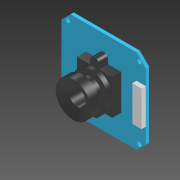
# Autodesk Inventor part: Arducam
Saved by Autodesk Inventor 2020 (Build 240168000, 168)
## iProperties
Created: 2020-11-17
Part Number: Arducam
Material: Generic
Document SubType Name: Modeling
Designer: valer
Density: 1 g/cm^3
Appearance: Default
Author: valer
Autodesk Inventor part; units mm, degrees
sketch "Base" plane through (0, 0, 0) normal (0, 0, 1) x (1, 0, 0)
  line L0 (-20.125, 20.125) -> (20.125, 20.125)
  line L1 (20.125, 20.125) -> (20.125, -20.125)
  line L2 (20.125, -20.125) -> (-20.125, -20.125)
  line L3 (-20.125, -20.125) -> (-20.125, 20.125)
  line L4 (-15.74, 20.125) -> (-20.125, 15.74)
  line L5 (15.74, 20.125) -> (20.125, 15.74)
  line L6 (-17.02, 17.02) -> (17.02, 17.02) construction
  line L7 (17.02, 17.02) -> (17.02, -17.02) construction
  line L8 (17.02, -17.02) -> (-17.02, -17.02) construction
  line L9 (-17.02, -17.02) -> (-17.02, 17.02) construction
  line L10 (-17.02, 17.02) -> (17.02, -17.02) construction
  line L11 (17.02, 17.02) -> (-17.02, -17.02) construction
  circle A0 centre (0, 0) radius 8.4
  circle A1 centre (17.02, 17.02) radius 1.05
  circle A2 centre (-17.02, 17.02) radius 1.05
  circle A3 centre (-17.02, -17.02) radius 1.05
  circle A4 centre (17.02, -17.02) radius 1.05
  line L12 (-20.125, -15.74) -> (-15.74, -20.125)
  line L13 (20.125, -15.74) -> (15.74, -20.125)
  point P0 (0, 0)
  point P1 (0, 0)
  dimension "d0" = 40.25
  dimension "d1" = 40.25
  dimension "d2" = 135
  dimension "d3" = 135
  dimension "d4" = 31.48
  dimension "d5" = 34.04
  dimension "d6" = 3.105
  dimension "d7" = 3.105
  dimension "d8" = 3.105
  dimension "d9" = 3.105
  dimension "d10" = 16.8
  dimension "d11" = 2.1
  dimension "d12" = 135
  dimension "d13" = 135
  dimension "d14" = 31.48
  dimension "d15" = 34.04
  dimension "d16" = 31.48
  constraints: 28 end point, 8 point on line, 5 centre point, 5 coincident, 5 perpendicular, 4 parallel, 3 equal radius, 2 horizontal, 2 midpoint
  measures "d0" distance of L0.start L0.end
  measures "d1" distance of L2.end L0.start
  measures "d2" angle of L0 L4
  measures "d3" angle of L0 L5
  measures "d4" distance of L5.start L4.start
  measures "d5" distance of L6.start L6.end
  measures "d6" distance between parallel lines of L3 L9
  measures "d7" distance between parallel lines of L1 L7
  measures "d8" distance between parallel lines of L0 L6
  measures "d9" distance between parallel lines of L2 L8
  measures "d10" diameter of A0
  measures "d11" diameter of A1
  measures "d12" angle of L2 L12
  measures "d13" angle of L2 L13
  measures "d14" distance of L12.start L4.end
  measures "d15" distance of L8.end L6.start
  measures "d16" distance of L13.start L5.end
extrude "BaseFeature" add sketch "Base" along normal blind 1.5 contours L0 L5 L1 L13 L2 L12 L3 L4 | A0
extrude "CameraFeature" add sketch "Base" along normal blind 16 contours A0
sketch "Sketch2" plane through (0, 0, 16) normal (0, 0, 1) x (1, 0, 0)
  circle A0 centre (0, 0) radius 8.4 projected
  circle A1 centre (0, 0) radius 4
  point P0 (0, 0)
  dimension "d28" = 8
  constraints: 1 centre point
  measures "d28" diameter of A1
extrude "Extrusion3" cut sketch "Sketch2" against normal blind 7.62 contours A1
sketch "Sketch4" plane through (0, 0, 1.5) normal (0, 0, 1) x (1, 0, 0)
  circle A0 centre (0, 0) radius 4 projected
  circle A1 centre (0, 0) radius 8.4 projected
  line L0 (-8.4, -8.4) -> (8.4, -8.4)
  line L1 (8.4, -8.4) -> (8.4, 8.4)
  line L2 (8.4, 8.4) -> (-8.4, 8.4)
  line L3 (-8.4, 8.4) -> (-8.4, -8.4)
  circle A2 centre (0, 0) radius 8.4 projected
  point P0 (0, 0)
  constraints: 8 end point, 4 tangent, 2 parallel, 1 horizontal, 1 perpendicular
extrude "Extrusion5" add sketch "Sketch4" along normal blind 4.32 contours A0 | A1 | L1 L0 A1 | A1 L2 L1 | A1 L3 L2 | L0 L3 A1
ref_plane "Work Plane1" through (0, 0, 7.82) normal (0, 0, 1) x (1, 0, 0)
ref_plane "Work Plane2" through (0, 0, 11.74) normal (0, 0, 1) x (1, 0, 0)
sketch "Sketch5" plane through (0, 0, 7.82) normal (0, 0, 1) x (1, 0, 0)
  circle A0 centre (0, 0) radius 8.4 projected
  circle A1 centre (0, 0) radius 5.64
  point P0 (0, 0)
  dimension "d33" = 11.28
  constraints: 1 centre point, 1 coincident
  measures "d33" diameter of A1
extrude "Extrusion6" cut sketch "Sketch5" along normal up to surface (3.92 mm away)
ref_plane "Work Plane3" through (0, 0, 14) normal (0, 0, 1) x (1, 0, 0)
sketch "Sketch6" plane through (0, 0, 16) normal (0, 0, 1) x (1, 0, 0)
  circle A0 centre (0, 0) radius 8.4 projected
  point P0 (0, 0)
sketch "Sketch7" plane through (0, 0, 14) normal (0, 0, 1) x (1, 0, 0)
  circle A0 centre (0, 0) radius 4 projected
  point P0 (0, 0)
loft "Loft1" cut profiles "Sketch7" section 2 edges at (-8.4, 0, 16)
sketch "Sketch8" plane through (0, 0, 1.5) normal (0, 0, 1) x (1, 0, 0)
  line L0 (8.4, 8.4) -> (0, 8.4) projected
  line L1 (0, 8.4) -> (-8.4, 8.4) projected
  line L2 (0, -8.4) -> (8.4, -8.4) projected
  line L3 (-8.4, -8.4) -> (0, -8.4) projected
  line L4 (15.74, 20.125) -> (-15.74, 20.125) construction
  line L5 (0, 20.125) -> (0, 8.4) construction
  line L6 (0, -8.4) -> (0, -20.125) construction
  line L7 (-15.74, -20.125) -> (15.74, -20.125) construction
  circle A0 centre (0, 10.4) radius 2.12
  line L8 (2.12, 10.4) -> (-2.12, 10.4) construction
  line L9 (-2.12, 10.4) -> (-2.12, 8.4)
  line L10 (-2.12, 8.4) -> (2.12, 8.4)
  line L11 (2.12, 8.4) -> (2.12, 10.4)
  line L12 (-28.175, 0) -> (28.175, 0) projected
  circle A1 centre (0, -10.4) radius 2.12
  line L13 (-2.12, -10.4) -> (-2.12, -8.4)
  line L14 (-2.12, -8.4) -> (2.12, -8.4)
  line L15 (2.12, -8.4) -> (2.12, -10.4)
  point P0 (0, 0)
  dimension "d41" = 4.24
  dimension "d42" = 2
  constraints: 18 end point, 5 symmetric about line, 4 point on circle, 2 centre point, 2 midpoint, 2 parallel, 2 perpendicular, 1 collinear, 1 horizontal, 1 point on line, 1 tangent, 1 other
  measures "d41" diameter of A0
  measures "d42" distance between parallel lines of L0 L8
extrude "Extrusion7" add sketch "Sketch8" along normal blind 4.32 contours L0 A0 L11 | L0 L1 A0 | L1 L9 A0 | L2 A1 L3 | L2 L15 A1 | A1 L13 L3 picked at (0, 11.1364) picked at (0, -11.1364)
sketch "Sketch9" plane through (0, 0, 1.5) normal (0, 0, 1) x (1, 0, 0)
  line L0 (20.06, 8.4) -> (15.7, 8.4)
  line L1 (15.7, 8.4) -> (15.7, -8.4)
  line L2 (15.7, -8.4) -> (20.06, -8.4)
  line L3 (20.06, -8.4) -> (20.06, 8.4)
  line L4 (8.4, 8.4) -> (2.12, 8.4) projected
  line L5 (2.12, -8.4) -> (8.4, -8.4) projected
  line L6 (8.4, -8.4) -> (8.4, 0) projected
  point P0 (0, 0)
  dimension "d45" = 4.36
  dimension "d46" = 7.3
  constraints: 8 end point, 2 collinear, 2 parallel, 1 horizontal, 1 perpendicular
  measures "d45" distance of L0.start L0.end
  measures "d46" distance between parallel lines of L1 L6
extrude "Extrusion8" add sketch "Sketch9" along normal blind 2
equation "\"d1\" = d0"
equation "\"d3\" = d2"
equation "\"d7\" = d6"
equation "\"d9\" = d8"
equation "\"d12\" = d2"
equation "\"d13\" = d2"
equation "\"d14\" = d4"
body "Solid1"
